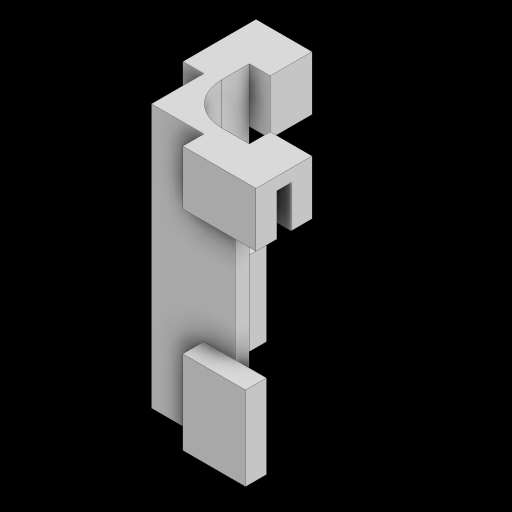
# Autodesk Inventor part: Codo
Saved by Autodesk Inventor 2024.2 (Build 282272000, 272)
## iProperties
Created: 2024-09-26
Part Number: Codo
Material: Generic
Document SubType Name: Modeling
Designer: jrcer
Density: 1 g/cm^3
Appearance: Default
Author: jrcer
Autodesk Inventor part; units mm, degrees
ref_plane "YZ Plane" through (0, 0, 0) normal (1, 0, 0) x (0, 1, 0)
ref_plane "XZ Plane" through (0, 0, 0) normal (0, 1, 0) x (-1, 0, 0)
ref_plane "XY Plane" through (0, 0, 0) normal (0, 0, 1) x (1, 0, 0)
sketch "Sketch2" plane through (0, 0, 0) normal (0, 1, 0) x (-1, 0, 0)
  line L0 (0, 0) -> (0, -20)
  line L1 (0, -20) -> (-3.4, -20)
  line L2 (-3.4, -20) -> (-3.4, -3.4)
  line L3 (-3.4, -3.4) -> (-20, -3.4)
  line L4 (-20, -3.4) -> (-20, 0)
  line L5 (-20, 0) -> (0, 0)
  dimension "d0" = 20
  dimension "d1" = 3.4
  constraints: 12 end point, 6 perpendicular, 1 horizontal, 1 vertical
  measures "d0" distance of L0.start L0.end
  measures "d1" distance of L0.end L1.end
extrude "Extrusion1" add sketch "Sketch2" along normal blind 63
sketch "Sketch3" plane through (0, 0, 0) normal (0, 0, 1) x (1, 0, 0)
  line L0 (20, 0) -> (20, 63) construction
  line L1 (12.5, 20) -> (27.5, 20)
  line L2 (27.5, 20) -> (27.5, 0)
  line L3 (27.5, 0) -> (12.5, 0)
  line L4 (12.5, 0) -> (12.5, 20)
  line L5 (12.5, 20) -> (27.5, 0) construction
  line L6 (27.5, 20) -> (12.5, 0) construction
  line L7 (0, 0) -> (20, 0) construction
  point P0 (20, 10)
  dimension "d4" = 15
  dimension "d5" = 20
  constraints: 12 end point, 2 midpoint, 2 parallel, 1 collinear, 1 horizontal, 1 perpendicular, 1 point on line
  measures "d4" distance of L2.end L3.end
  measures "d5" distance of L1.end L2.end
extrude "Extrusion2" add sketch "Sketch3" along normal blind 5
sketch "Sketch4" plane through (0, 0, -20) normal (-1, 0, 0) x (0, 0, 1)
  line L0 (0, 0) -> (0, 63) construction
  line L1 (0, 0) -> (20, 0) construction
  line L2 (-7.5, 20) -> (7.5, 20)
  line L3 (7.5, 20) -> (7.5, 0)
  line L4 (7.5, 0) -> (-7.5, 0)
  line L5 (-7.5, 0) -> (-7.5, 20)
  line L6 (-7.5, 20) -> (7.5, 0) construction
  line L7 (7.5, 20) -> (-7.5, 0) construction
  point P0 (0, 10)
  dimension "d8" = 15
  dimension "d9" = 20
  constraints: 12 end point, 2 midpoint, 2 parallel, 1 collinear, 1 horizontal, 1 perpendicular, 1 point on line
  measures "d8" distance of L3.end L4.end
  measures "d9" distance of L2.end L3.end
extrude "Extrusion3" add sketch "Sketch4" along normal blind 5
fillet "Face Fillet1" radius 10 1 edges at (3.4, 31.5, -3.4)
sketch "Sketch5" plane through (0, 63, 0) normal (0, 1, 0) x (1, 0, 0)
  line L0 (8.4, 20) -> (3.4, 20)
  line L1 (3.4, 20) -> (3.4, 30)
  line L2 (3.4, 30) -> (8.4, 30)
  line L3 (8.4, 30) -> (8.4, 20)
  line L4 (8.4, 20) -> (3.4, 30) construction
  line L5 (3.4, 20) -> (8.4, 30) construction
  line L6 (30, 3.4) -> (20, 3.4)
  line L7 (20, 3.4) -> (20, 8.4)
  line L8 (20, 8.4) -> (30, 8.4)
  line L9 (30, 8.4) -> (30, 3.4)
  line L10 (30, 3.4) -> (20, 8.4) construction
  line L11 (20, 3.4) -> (30, 8.4) construction
  line L12 (3.4, 20) -> (0, 20) construction
  line L13 (20, 3.4) -> (13.4, 3.4) construction
  line L14 (3.4, 13.4) -> (3.4, 20) construction
  line L15 (0, 12.5) -> (-5, 12.5) construction
  line L16 (12.5, 0) -> (12.5, -5) construction
  line L17 (-5, 12.5) -> (-5, 27.5) projected
  line L18 (-5, 12.5) -> (0, 12.5)
  line L19 (0, 12.5) -> (0, 30)
  line L20 (0, 30) -> (-5, 30)
  line L21 (-5, 30) -> (-5, 12.5)
  line L22 (12.5, 0) -> (30, 0)
  line L23 (30, 0) -> (30, -5)
  line L24 (30, -5) -> (12.5, -5)
  line L25 (12.5, -5) -> (12.5, 0)
  point P0 (5.9, 25)
  point P1 (25, 5.9)
  point P2 (20, 0)
  dimension "d20" = 5
  dimension "d21" = 10
  dimension "d22" = 10
  dimension "d23" = 5
  constraints: 40 end point, 8 parallel, 5 collinear, 4 horizontal, 4 midpoint, 4 perpendicular, 2 equal length
  measures "d20" distance of L1.end L2.end
  measures "d21" distance of L0.end L1.end
  measures "d22" distance of L7.end L8.end
  measures "d23" distance of L6.end L7.end
extrude "Extrusion4" add sketch "Sketch5" against normal blind 13
sketch "Sketch6" plane through (3.4, 0, -20) normal (0, 0, -1) x (-1, 0, 0)
  line L0 (0, 63) -> (3.4, 63) construction
  line L1 (0, 63) -> (0, 50) construction
  line L2 (3.4, 63) -> (3.4, 50) construction
  line L3 (0, 63) -> (3.4, 63)
  line L4 (3.4, 63) -> (3.4, 60)
  line L5 (3.4, 60) -> (0, 60)
  line L6 (0, 60) -> (0, 63)
  line L7 (0, 63) -> (3.4, 60) construction
  line L8 (3.4, 63) -> (0, 60) construction
  point P0 (3.4, 0)
  point P1 (1.7, 61.5)
  dimension "d25" = 3.4
  dimension "d26" = 3
  constraints: 12 end point, 2 midpoint, 2 parallel, 1 collinear, 1 horizontal, 1 perpendicular
  measures "d25" distance of L4.end L5.end
  measures "d26" distance of L3.end L4.end
extrude "Extrusion5" add sketch "Sketch6" along normal blind 10
sketch "Sketch7" plane through (20, 0, 0) normal (1, 0, 0) x (0, 0, -1)
  line L0 (0, 63) -> (3.4, 63) construction
  line L1 (0, 63) -> (0, 50) construction
  line L2 (3.4, 63) -> (3.4, 50) construction
  line L3 (0, 63) -> (3.4, 63)
  line L4 (3.4, 63) -> (3.4, 60)
  line L5 (3.4, 60) -> (0, 60)
  line L6 (0, 60) -> (0, 63)
  line L7 (0, 63) -> (3.4, 60) construction
  line L8 (3.4, 63) -> (0, 60) construction
  point P0 (0, 0)
  point P1 (1.7, 61.5)
  point P2 (1.7, 63)
  dimension "d29" = 3.4
  dimension "d30" = 3
  constraints: 12 end point, 3 midpoint, 2 parallel, 1 collinear, 1 horizontal, 1 perpendicular, 1 vertical alignment
  measures "d29" distance of L4.end L5.end
  measures "d30" distance of L3.end L4.end
extrude "Extrusion6" add sketch "Sketch7" along normal blind 10
body "Solid1"
